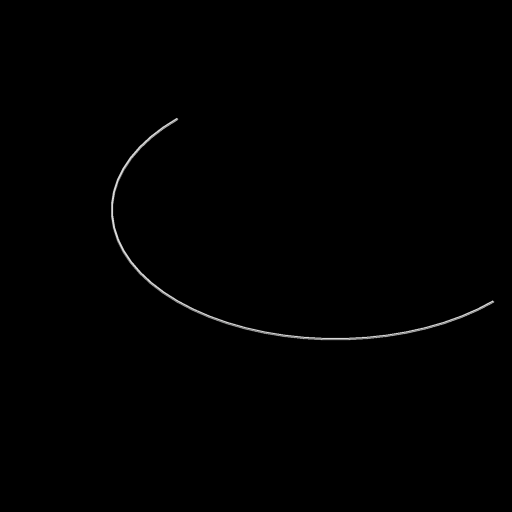
# Autodesk Inventor part: R1M
Saved by Autodesk Inventor 2024.2 (Build 282272000, 272)
## iProperties
Created: 2024-10-01
Part Number: R1M
Material: Generic
Document SubType Name: Modeling
Designer: jrcer
Density: 1 g/cm^3
Appearance: Default
Author: jrcer
Autodesk Inventor part; units mm, degrees
ref_plane "YZ Plane" through (0, 0, 0) normal (1, 0, 0) x (0, 1, 0)
ref_plane "XZ Plane" through (0, 0, 0) normal (0, 1, 0) x (-1, 0, 0)
ref_plane "XY Plane" through (0, 0, 0) normal (0, 0, 1) x (1, 0, 0)
sketch "Sketch1" plane through (0, 0, 0) normal (0, 1, 0) x (-1, 0, 0)
  circle A0 centre (0, 0) radius 500
  circle A1 centre (0, 0) radius 505
  line L0 (505, 0) -> (500, 0)
  line L1 (-505, 0) -> (-500, 0)
  point P0 (502.5, 0)
  point P1 (-502.5, 0)
  dimension "d0" = 1000
  dimension "d1" = 1010
  constraints: 4 end point, 4 point on circle, 2 centre point, 2 coincident, 2 horizontal, 2 horizontal alignment, 2 midpoint
  measures "d0" diameter of A0
  measures "d1" diameter of A1
extrude "Extrusion1" add sketch "Sketch1" along normal blind 3 contours A0 L1 A1 L0 picked at (-373.9076, 336.623)
body "Solid1"
